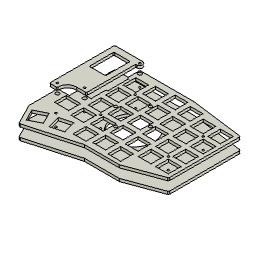
Sofle_pico_v3.4_Acrylic_case v20 (Autodesk Fusion 360 design; units mm, degrees)
Autodesk Fusion 360 part; units mm, degrees
sketch "OLED_raw_import" plane through (0, 0, 0) normal (0, 0, 1) x (1, 0, 0)
  arc A0 (31.596, -60.3171) -> (30.596, -61.3171) centre (30.596, -60.3171) cw
  arc A1 (3.2145, -72.447) -> (2.2145, -71.447) centre (3.2146, -71.4469) cw
  line L0 (31.596, -60.3171) -> (31.596, -7.2074)
  arc A2 (2.1895, -2.4227) -> (3.6899, -0.9223) centre (3.69, -2.4228) cw
  line L1 (2.2145, -71.447) -> (2.1895, -2.4227)
  arc A3 (10.656, -71.447) -> (9.656, -72.447) centre (9.656, -71.447) cw
  line L2 (31.596, -7.2074) -> (32.7961, -7.2077)
  line L3 (3.6899, -0.9224) -> (32.7961, -0.9224)
  line L4 (9.656, -72.447) -> (3.2145, -72.447)
  line L5 (20.846, -61.3171) -> (30.596, -61.3171)
  arc A4 (10.656, -71.447) -> (20.8461, -61.3171) centre (20.7861, -71.447) cw
  arc A5 (32.7961, -0.9224) -> (32.7961, -7.2074) centre (32.7783, -4.0649) cw
  circle A6 centre (32.7961, -4.0649) radius 1.1
  circle A7 centre (25.926, -57.5371) radius 1.1
  circle A8 centre (6.4353, -67.947) radius 1.1
  line L6 (-6.3855, 6.3482) -> (54.659, 6.3482)
  line L7 (54.659, 6.3482) -> (54.659, -85.336)
  line L8 (54.659, -85.336) -> (-6.3855, -85.336)
  line L9 (-6.3855, -85.336) -> (-6.3855, 6.3482)
  line L10 (32.7961, -0.9224) -> (32.7961, 6.3482)
  line L11 (32.7961, -7.2077) -> (54.659, -7.2077)
  line L12 (32.7961, -0.9224) -> (54.659, -1.0458)
  line L13 (3.6899, -0.9224) -> (3.6899, 6.3482)
  line L14 (2.1895, -2.4227) -> (-6.3855, -2.4227)
  line L15 (2.2145, -71.447) -> (-6.3855, -71.447)
  line L16 (3.2145, -72.447) -> (3.2145, -85.336)
  line L17 (9.656, -72.447) -> (9.656, -85.336)
  line L18 (10.656, -71.447) -> (54.659, -71.447)
  line L19 (30.596, -61.3171) -> (30.596, -71.447)
  line L20 (31.596, -60.3171) -> (54.659, -60.3171)
  line L21 (32.7961, -7.2074) -> (32.7961, -60.3171)
  point P0 (33.8961, -4.0649)
  point P1 (27.026, -57.5371)
  point P2 (7.5352, -67.947)
  constraint horizontal L6
  constraint vertical L7
  constraint horizontal L8
  constraint vertical L9
  constraint coincident L6 L10.end
  constraint perpendicular L6 L10
  constraint coincident L7 L11.end
  constraint perpendicular L7 L11
  constraint coincident L7 L12.end
  constraint tangent A5 L12
  constraint coincident L6 L13.end
  constraint perpendicular L6 L13
  constraint coincident L9 L14.end
  constraint perpendicular L9 L14
  constraint coincident L9 L15.end
  constraint perpendicular L9 L15
  constraint coincident L8 L16.end
  constraint perpendicular L8 L16
  constraint coincident L8 L17.end
  constraint perpendicular L8 L17
  constraint coincident L7 L18.end
  constraint perpendicular L7 L18
  constraint coincident L18 L19.end
  constraint perpendicular L18 L19
  constraint coincident L7 L20.end
  constraint perpendicular L7 L20
  constraint coincident L20 L21.end
  constraint perpendicular L20 L21
extrude "Extrude1" add sketch "OLED_raw_import" along normal blind 3 contours A0 A1 L0 A2 L1 A3 L2 L3 L4 L5 A4 A5 makes body 1
sketch "sofle_pico_OLED_v3.4" plane through (0, 0, 3) normal (0, 0, 1) x (-1, 0, 0)
  circle A0 centre (-25.926, 57.5371) radius 1.1
  circle A1 centre (-32.7961, 4.0649) radius 1.1
  circle A2 centre (-6.4353, 67.947) radius 1.1
  line L0 (-3.6899, 0.9224) -> (-3.6899, 0.9223)
  arc A3 (-3.6899, 0.9223) -> (-2.1895, 2.4227) centre (-3.69, 2.4228) ccw
  line L1 (-2.1895, 2.4227) -> (-2.2145, 71.447)
  arc A4 (-2.2145, 71.447) -> (-3.2145, 72.447) centre (-3.2146, 71.4469) ccw
  line L2 (-3.2145, 72.447) -> (-9.656, 72.447)
  arc A5 (-9.656, 72.447) -> (-10.656, 71.447) centre (-9.656, 71.447) ccw
  arc A6 (-20.8461, 61.3171) -> (-10.656, 71.447) centre (-20.7861, 71.447) ccw
  line L3 (-20.8461, 61.3171) -> (-30.596, 61.3171)
  arc A7 (-30.596, 61.3171) -> (-31.596, 60.3171) centre (-30.596, 60.3171) ccw
  line L4 (-31.596, 60.3171) -> (-31.596, 7.2074)
  line L5 (-31.596, 7.2074) -> (-32.7961, 7.2077)
  line L6 (-32.7961, 7.2077) -> (-32.7961, 7.2074)
  arc A8 (-32.7961, 7.2074) -> (-32.7961, 0.9224) centre (-32.7783, 4.0649) ccw
  line L7 (-32.7961, 0.9224) -> (-3.6899, 0.9224)
sketch "keyplate_raw_import" plane through (0, 0, 0) normal (0, 0, 1) x (1, 0, 0)
  arc A0 (64.0629, -94.1892) -> (63.8994, -93.4815) centre (65.4011, -93.5073) cw
  line L0 (64.0629, -94.1892) -> (74.8738, -115.4059)
  arc A1 (91.5088, -0.9271) -> (92.5088, 0.0729) centre (92.5088, -0.9271) cw
  line L1 (150.6703, 0.0729) -> (207.9837, -7.326)
  arc A2 (92.5088, -13.8721) -> (91.5088, -12.8721) centre (92.5088, -12.8721) cw
  line L2 (91.5088, -37.8219) -> (91.5088, -53.3818)
  line L3 (92.5088, -13.8721) -> (93.2959, -13.8721)
  line L4 (63.8994, -63.3988) -> (63.8994, -93.4815)
  line L5 (150.6703, 0.0729) -> (92.5088, 0.0729)
  line L6 (76.596, -62.3988) -> (76.596, -53.3818)
  arc A3 (207.9837, -7.326) -> (209.3199, -8.827) centre (207.8088, -8.827) cw
  line L7 (92.5088, -36.8219) -> (93.2959, -36.8219)
  line L8 (93.2959, -36.8219) -> (93.2959, -13.8721)
  line L9 (91.5088, -53.3818) -> (76.596, -53.3818)
  line L10 (169.7202, -100.6763) -> (208.4142, -86.4036)
  line L11 (209.3199, -8.827) -> (209.3199, -85.0265)
  line L12 (131.6205, -100.6763) -> (169.7202, -100.6763)
  line L13 (91.5088, -0.9271) -> (91.5088, -12.8721)
  line L14 (64.8994, -62.3988) -> (76.596, -62.3988)
  arc A4 (76.6062, -116.1717) -> (74.8738, -115.4059) centre (76.2102, -114.725) cw
  arc A5 (209.3199, -85.0265) -> (208.4142, -86.4037) centre (207.8201, -85.0266) cw
  line L15 (76.6062, -116.1717) -> (131.6205, -100.6763)
  arc A6 (91.5088, -37.8219) -> (92.5088, -36.8219) centre (92.5088, -37.8219) cw
  arc A7 (63.8994, -63.3988) -> (64.8994, -62.3988) centre (64.8994, -63.3988) cw
  line L16 (90.4959, -76.9516) -> (74.896, -76.9516)
  line L17 (74.896, -76.9516) -> (74.896, -63.9517)
  line L18 (74.896, -63.9517) -> (90.4959, -63.9517)
  line L19 (90.4959, -63.9517) -> (90.4959, -76.9516)
  circle A8 centre (188.7852, -27.862) radius 1.1
  circle A9 centre (188.7703, -65.9767) radius 1.1
  circle A10 centre (111.9358, -25.462) radius 1.1
  circle A11 centre (112.0257, -63.4117) radius 1.1
  circle A12 centre (112.5707, -47.3218) radius 1.75
  circle A13 centre (131.6206, -28.272) radius 1.75
  circle A14 centre (131.6206, -66.3717) radius 1.75
  circle A15 centre (150.6704, -47.3218) radius 1.75
  circle A16 centre (86.0859, -86.4815) radius 1.1
  circle A17 centre (94.5059, -3.0695) radius 2.05
  circle A18 centre (87.6359, -56.5418) radius 2.05
  circle A19 centre (68.1451, -66.9517) radius 2.05
  line L20 (110.0457, -22.952) -> (96.0458, -22.952)
  line L21 (96.0458, -22.952) -> (96.0458, -8.9521)
  line L22 (96.0458, -8.9521) -> (110.0457, -8.9521)
  line L23 (110.0457, -8.9521) -> (110.0457, -22.952)
  line L24 (148.1456, -17.952) -> (134.1457, -17.952)
  line L25 (134.1457, -17.952) -> (134.1457, -3.9521)
  line L26 (134.1457, -3.9521) -> (148.1456, -3.9521)
  line L27 (148.1456, -3.9521) -> (148.1456, -17.952)
  line L28 (110.0457, -61.0517) -> (96.0458, -61.0517)
  line L29 (96.0458, -61.0517) -> (96.0458, -47.0518)
  line L30 (96.0458, -47.0518) -> (110.0457, -47.0518)
  line L31 (110.0457, -47.0518) -> (110.0457, -61.0517)
  line L32 (129.0957, -58.5517) -> (115.0957, -58.5517)
  line L33 (115.0957, -58.5517) -> (115.0957, -44.5518)
  line L34 (115.0957, -44.5518) -> (129.0957, -44.5518)
  line L35 (129.0957, -44.5518) -> (129.0957, -58.5517)
  line L36 (148.1456, -75.1016) -> (134.1457, -75.1016)
  line L37 (134.1457, -75.1016) -> (134.1457, -61.1017)
  line L38 (134.1457, -61.1017) -> (148.1456, -61.1017)
  line L39 (148.1456, -61.1017) -> (148.1456, -75.1016)
  line L40 (186.2452, -82.5016) -> (172.2453, -82.5016)
  line L41 (172.2453, -82.5016) -> (172.2453, -68.5017)
  line L42 (172.2453, -68.5017) -> (186.2452, -68.5017)
  line L43 (186.2452, -68.5017) -> (186.2452, -82.5016)
  line L44 (76.2327, -109.2072) -> (69.8768, -96.7332)
  line L45 (69.8768, -96.7332) -> (82.3508, -90.3773)
  line L46 (82.3508, -90.3773) -> (88.7067, -102.8513)
  line L47 (88.7067, -102.8513) -> (76.2327, -109.2072)
  line L48 (108.669, -99.3012) -> (95.1461, -102.9246)
  line L49 (95.1461, -102.9246) -> (91.5227, -89.4018)
  line L50 (91.5227, -89.4018) -> (105.0456, -85.7783)
  line L51 (105.0456, -85.7783) -> (108.669, -99.3012)
  line L52 (205.2951, -44.4018) -> (191.2952, -44.4018)
  line L53 (191.2952, -44.4018) -> (191.2952, -30.4019)
  line L54 (191.2952, -30.4019) -> (205.2951, -30.4019)
  line L55 (205.2951, -30.4019) -> (205.2951, -44.4018)
  line L56 (205.2951, -63.4517) -> (191.2952, -63.4517)
  line L57 (191.2952, -63.4517) -> (191.2952, -49.4518)
  line L58 (191.2952, -49.4518) -> (205.2951, -49.4518)
  line L59 (205.2951, -49.4518) -> (205.2951, -63.4517)
  line L60 (205.2951, -82.5016) -> (191.2952, -82.5016)
  line L61 (191.2952, -82.5016) -> (191.2952, -68.5017)
  line L62 (191.2952, -68.5017) -> (205.2951, -68.5017)
  line L63 (205.2951, -68.5017) -> (205.2951, -82.5016)
  line L64 (167.1953, -20.452) -> (153.1954, -20.452)
  line L65 (153.1954, -20.452) -> (153.1954, -6.4521)
  line L66 (153.1954, -6.4521) -> (167.1953, -6.4521)
  line L67 (167.1953, -6.4521) -> (167.1953, -20.452)
  line L68 (186.2452, -25.352) -> (172.2453, -25.352)
  line L69 (172.2453, -25.352) -> (172.2453, -11.3521)
  line L70 (172.2453, -11.3521) -> (186.2452, -11.3521)
  line L71 (186.2452, -11.3521) -> (186.2452, -25.352)
  line L72 (129.0957, -39.5019) -> (115.0957, -39.5019)
  line L73 (115.0957, -39.5019) -> (115.0957, -25.502)
  line L74 (115.0957, -25.502) -> (129.0957, -25.502)
  line L75 (129.0957, -25.502) -> (129.0957, -39.5019)
  line L76 (167.1953, -39.5019) -> (153.1954, -39.5019)
  line L77 (153.1954, -39.5019) -> (153.1954, -25.502)
  line L78 (153.1954, -25.502) -> (167.1953, -25.502)
  line L79 (167.1953, -25.502) -> (167.1953, -39.5019)
  line L80 (148.1456, -37.0019) -> (134.1457, -37.0019)
  line L81 (134.1457, -37.0019) -> (134.1457, -23.002)
  line L82 (134.1457, -23.002) -> (148.1456, -23.002)
  line L83 (148.1456, -23.002) -> (148.1456, -37.0019)
  line L84 (167.1953, -58.5517) -> (153.1954, -58.5517)
  line L85 (153.1954, -58.5517) -> (153.1954, -44.5518)
  line L86 (153.1954, -44.5518) -> (167.1953, -44.5518)
  line L87 (167.1953, -44.5518) -> (167.1953, -58.5517)
  line L88 (205.2951, -25.352) -> (191.2952, -25.352)
  line L89 (191.2952, -25.352) -> (191.2952, -11.3521)
  line L90 (191.2952, -11.3521) -> (205.2951, -11.3521)
  line L91 (205.2951, -11.3521) -> (205.2951, -25.352)
  line L92 (110.0457, -42.0019) -> (96.0458, -42.0019)
  line L93 (96.0458, -42.0019) -> (96.0458, -28.002)
  line L94 (96.0458, -28.002) -> (110.0457, -28.002)
  line L95 (110.0457, -28.002) -> (110.0457, -42.0019)
  line L96 (167.1953, -96.6515) -> (153.1954, -96.6515)
  line L97 (153.1954, -96.6515) -> (153.1954, -82.6516)
  line L98 (153.1954, -82.6516) -> (167.1953, -82.6516)
  line L99 (167.1953, -82.6516) -> (167.1953, -96.6515)
  line L100 (186.2452, -44.4018) -> (172.2453, -44.4018)
  line L101 (172.2453, -44.4018) -> (172.2453, -30.4019)
  line L102 (172.2453, -30.4019) -> (186.2452, -30.4019)
  line L103 (186.2452, -30.4019) -> (186.2452, -44.4018)
  line L104 (167.1953, -77.6016) -> (153.1954, -77.6016)
  line L105 (153.1954, -77.6016) -> (153.1954, -63.6017)
  line L106 (153.1954, -63.6017) -> (167.1953, -63.6017)
  line L107 (167.1953, -63.6017) -> (167.1953, -77.6016)
  line L108 (186.2452, -63.4517) -> (172.2453, -63.4517)
  line L109 (172.2453, -63.4517) -> (172.2453, -49.4518)
  line L110 (172.2453, -49.4518) -> (186.2452, -49.4518)
  line L111 (186.2452, -49.4518) -> (186.2452, -63.4517)
  line L112 (148.1456, -94.1515) -> (134.1457, -94.1515)
  line L113 (134.1457, -94.1515) -> (134.1457, -80.1516)
  line L114 (134.1457, -80.1516) -> (148.1456, -80.1516)
  line L115 (148.1456, -80.1516) -> (148.1456, -94.1515)
  line L116 (148.1456, -56.0518) -> (134.1457, -56.0518)
  line L117 (134.1457, -56.0518) -> (134.1457, -42.0519)
  line L118 (134.1457, -42.0519) -> (148.1456, -42.0519)
  line L119 (148.1456, -42.0519) -> (148.1456, -56.0518)
  line L120 (129.0957, -20.452) -> (115.0957, -20.452)
  line L121 (115.0957, -20.452) -> (115.0957, -6.4521)
  line L122 (115.0957, -6.4521) -> (129.0957, -6.4521)
  line L123 (129.0957, -6.4521) -> (129.0957, -20.452)
  line L124 (129.0957, -77.6016) -> (115.0957, -77.6016)
  line L125 (115.0957, -77.6016) -> (115.0957, -63.6017)
  line L126 (115.0957, -63.6017) -> (129.0957, -63.6017)
  line L127 (129.0957, -63.6017) -> (129.0957, -77.6016)
  line L128 (129.0957, -96.6515) -> (115.0957, -96.6515)
  line L129 (115.0957, -96.6515) -> (115.0957, -82.6516)
  line L130 (115.0957, -82.6516) -> (129.0957, -82.6516)
  line L131 (129.0957, -82.6516) -> (129.0957, -96.6515)
  line L132 (110.0457, -80.1016) -> (96.0458, -80.1016)
  line L133 (96.0458, -80.1016) -> (96.0458, -66.1017)
  line L134 (96.0458, -66.1017) -> (110.0457, -66.1017)
  line L135 (110.0457, -66.1017) -> (110.0457, -80.1016)
  line L136 (58.3963, 5.3223) -> (215.5932, 5.3223)
  line L137 (215.5932, 5.3223) -> (215.5932, -121.9444)
  line L138 (215.5932, -121.9444) -> (58.3963, -121.9444)
  line L139 (58.3963, -121.9444) -> (58.3963, 5.3223)
  line L140 (76.6062, -116.1717) -> (76.6062, -121.9444)
  line L141 (131.6205, -100.6763) -> (131.6205, -121.9444)
  line L142 (209.3199, -8.827) -> (215.5932, -8.827)
  line L143 (207.9837, -7.326) -> (207.9837, 5.3223)
  line L144 (91.5088, -12.8721) -> (58.3963, -12.8721)
  line L145 (92.5088, 0.0729) -> (92.5088, 5.3223)
  line L146 (76.596, -53.3818) -> (58.3963, -53.3818)
  line L147 (209.3199, -85.0265) -> (215.5932, -85.0265)
  line L148 (208.4142, -86.4037) -> (215.5932, -86.4037)
  line L149 (169.7202, -100.6763) -> (169.7202, -121.9444)
  line L150 (208.4142, -86.4036) -> (208.4142, -121.9444)
  point P0 (189.8851, -27.862)
  point P1 (189.8702, -65.9767)
  point P2 (113.0358, -25.462)
  point P3 (113.1257, -63.4117)
  point P4 (114.3207, -47.3218)
  point P5 (133.3706, -28.272)
  point P6 (133.3706, -66.3717)
  point P7 (152.4204, -47.3218)
  point P8 (87.1859, -86.4815)
  point P9 (96.5559, -3.0695)
  point P10 (89.6859, -56.5418)
  point P11 (70.1951, -66.9517)
  constraint horizontal L136
  constraint vertical L137
  constraint horizontal L138
  constraint vertical L139
  constraint coincident L138 L140.end
  constraint perpendicular L138 L140
  constraint coincident L138 L141.end
  constraint perpendicular L138 L141
  constraint coincident L137 L142.end
  constraint perpendicular L137 L142
  constraint coincident L136 L143.end
  constraint perpendicular L136 L143
  constraint coincident L139 L144.end
  constraint perpendicular L139 L144
  constraint coincident L136 L145.end
  constraint perpendicular L136 L145
  constraint coincident L139 L146.end
  constraint perpendicular L139 L146
  constraint coincident L137 L147.end
  constraint perpendicular L137 L147
  constraint coincident L137 L148.end
  constraint perpendicular L137 L148
  constraint coincident L138 L149.end
  constraint perpendicular L138 L149
  constraint coincident L138 L150.end
  constraint perpendicular L138 L150
extrude "Extrude2" add sketch "keyplate_raw_import" along normal blind 3 separate body contours A0 L0 A1 L1 A2 L2 L3 L4 L5 L6 A3 L7 L8 L9 L10 L11 L12 L13 L14 A4 A5 L15 A6 A7 makes body 2
sketch "sofle_pico_keyplate_v3.4" plane through (0, 0, 3) normal (0, 0, 1) x (-1, 0, 0)
  line L0 (-74.896, 63.9517) -> (-90.4959, 63.9517)
  line L1 (-90.4959, 63.9517) -> (-90.4959, 76.9516)
  line L2 (-90.4959, 76.9516) -> (-74.896, 76.9516)
  line L3 (-74.896, 76.9516) -> (-74.896, 63.9517)
  circle A0 centre (-131.6206, 66.3717) radius 1.75
  circle A1 centre (-188.7852, 27.862) radius 1.1
  circle A2 centre (-188.7703, 65.9767) radius 1.1
  circle A3 centre (-111.9358, 25.462) radius 1.1
  circle A4 centre (-112.0257, 63.4117) radius 1.1
  line L4 (-172.2453, 11.3521) -> (-186.2452, 11.3521)
  line L5 (-186.2452, 11.3521) -> (-186.2452, 25.352)
  line L6 (-186.2452, 25.352) -> (-172.2453, 25.352)
  line L7 (-172.2453, 25.352) -> (-172.2453, 11.3521)
  circle A5 centre (-112.5707, 47.3218) radius 1.75
  circle A6 centre (-131.6206, 28.272) radius 1.75
  line L8 (-82.3508, 90.3773) -> (-88.7067, 102.8513)
  line L9 (-88.7067, 102.8513) -> (-76.2327, 109.2072)
  line L10 (-76.2327, 109.2072) -> (-69.8768, 96.7332)
  line L11 (-69.8768, 96.7332) -> (-82.3508, 90.3773)
  line L12 (-91.5227, 89.4018) -> (-105.0456, 85.7783)
  line L13 (-105.0456, 85.7783) -> (-108.669, 99.3012)
  line L14 (-108.669, 99.3012) -> (-95.1461, 102.9246)
  line L15 (-95.1461, 102.9246) -> (-91.5227, 89.4018)
  line L16 (-134.1457, 3.9521) -> (-148.1456, 3.9521)
  line L17 (-148.1456, 3.9521) -> (-148.1456, 17.952)
  line L18 (-148.1456, 17.952) -> (-134.1457, 17.952)
  line L19 (-134.1457, 17.952) -> (-134.1457, 3.9521)
  line L20 (-96.0458, 8.9521) -> (-110.0457, 8.9521)
  line L21 (-110.0457, 8.9521) -> (-110.0457, 22.952)
  line L22 (-110.0457, 22.952) -> (-96.0458, 22.952)
  line L23 (-96.0458, 22.952) -> (-96.0458, 8.9521)
  circle A7 centre (-68.1451, 66.9517) radius 2.05
  circle A8 centre (-87.6359, 56.5418) radius 2.05
  circle A9 centre (-94.5059, 3.0695) radius 2.05
  circle A10 centre (-86.0859, 86.4815) radius 1.1
  circle A11 centre (-150.6704, 47.3218) radius 1.75
  line L24 (-96.0458, 28.002) -> (-110.0457, 28.002)
  line L25 (-110.0457, 28.002) -> (-110.0457, 42.0019)
  line L26 (-110.0457, 42.0019) -> (-96.0458, 42.0019)
  line L27 (-96.0458, 42.0019) -> (-96.0458, 28.002)
  line L28 (-172.2453, 68.5017) -> (-186.2452, 68.5017)
  line L29 (-186.2452, 68.5017) -> (-186.2452, 82.5016)
  line L30 (-186.2452, 82.5016) -> (-172.2453, 82.5016)
  line L31 (-172.2453, 82.5016) -> (-172.2453, 68.5017)
  line L32 (-134.1457, 61.1017) -> (-148.1456, 61.1017)
  line L33 (-148.1456, 61.1017) -> (-148.1456, 75.1016)
  line L34 (-148.1456, 75.1016) -> (-134.1457, 75.1016)
  line L35 (-134.1457, 75.1016) -> (-134.1457, 61.1017)
  line L36 (-96.0458, 47.0518) -> (-110.0457, 47.0518)
  line L37 (-110.0457, 47.0518) -> (-110.0457, 61.0517)
  line L38 (-110.0457, 61.0517) -> (-96.0458, 61.0517)
  line L39 (-96.0458, 61.0517) -> (-96.0458, 47.0518)
  line L40 (-115.0957, 44.5518) -> (-129.0957, 44.5518)
  line L41 (-129.0957, 44.5518) -> (-129.0957, 58.5517)
  line L42 (-129.0957, 58.5517) -> (-115.0957, 58.5517)
  line L43 (-115.0957, 58.5517) -> (-115.0957, 44.5518)
  line L44 (-115.0957, 25.502) -> (-129.0957, 25.502)
  line L45 (-129.0957, 25.502) -> (-129.0957, 39.5019)
  line L46 (-129.0957, 39.5019) -> (-115.0957, 39.5019)
  line L47 (-115.0957, 39.5019) -> (-115.0957, 25.502)
  line L48 (-153.1954, 6.4521) -> (-167.1953, 6.4521)
  line L49 (-167.1953, 6.4521) -> (-167.1953, 20.452)
  line L50 (-167.1953, 20.452) -> (-153.1954, 20.452)
  line L51 (-153.1954, 20.452) -> (-153.1954, 6.4521)
  line L52 (-134.1457, 80.1516) -> (-148.1456, 80.1516)
  line L53 (-148.1456, 80.1516) -> (-148.1456, 94.1515)
  line L54 (-148.1456, 94.1515) -> (-134.1457, 94.1515)
  line L55 (-134.1457, 94.1515) -> (-134.1457, 80.1516)
  line L56 (-191.2952, 68.5017) -> (-205.2951, 68.5017)
  line L57 (-205.2951, 68.5017) -> (-205.2951, 82.5016)
  line L58 (-205.2951, 82.5016) -> (-191.2952, 82.5016)
  line L59 (-191.2952, 82.5016) -> (-191.2952, 68.5017)
  line L60 (-191.2952, 30.4019) -> (-205.2951, 30.4019)
  line L61 (-205.2951, 30.4019) -> (-205.2951, 44.4018)
  line L62 (-205.2951, 44.4018) -> (-191.2952, 44.4018)
  line L63 (-191.2952, 44.4018) -> (-191.2952, 30.4019)
  line L64 (-191.2952, 49.4518) -> (-205.2951, 49.4518)
  line L65 (-205.2951, 49.4518) -> (-205.2951, 63.4517)
  line L66 (-205.2951, 63.4517) -> (-191.2952, 63.4517)
  line L67 (-191.2952, 63.4517) -> (-191.2952, 49.4518)
  line L68 (-134.1457, 42.0519) -> (-148.1456, 42.0519)
  line L69 (-148.1456, 42.0519) -> (-148.1456, 56.0518)
  line L70 (-148.1456, 56.0518) -> (-134.1457, 56.0518)
  line L71 (-134.1457, 56.0518) -> (-134.1457, 42.0519)
  line L72 (-191.2952, 11.3521) -> (-205.2951, 11.3521)
  line L73 (-205.2951, 11.3521) -> (-205.2951, 25.352)
  line L74 (-205.2951, 25.352) -> (-191.2952, 25.352)
  line L75 (-191.2952, 25.352) -> (-191.2952, 11.3521)
  line L76 (-153.1954, 44.5518) -> (-167.1953, 44.5518)
  line L77 (-167.1953, 44.5518) -> (-167.1953, 58.5517)
  line L78 (-167.1953, 58.5517) -> (-153.1954, 58.5517)
  line L79 (-153.1954, 58.5517) -> (-153.1954, 44.5518)
  line L80 (-134.1457, 23.002) -> (-148.1456, 23.002)
  line L81 (-148.1456, 23.002) -> (-148.1456, 37.0019)
  line L82 (-148.1456, 37.0019) -> (-134.1457, 37.0019)
  line L83 (-134.1457, 37.0019) -> (-134.1457, 23.002)
  line L84 (-153.1954, 25.502) -> (-167.1953, 25.502)
  line L85 (-167.1953, 25.502) -> (-167.1953, 39.5019)
  line L86 (-167.1953, 39.5019) -> (-153.1954, 39.5019)
  line L87 (-153.1954, 39.5019) -> (-153.1954, 25.502)
  line L88 (-172.2453, 49.4518) -> (-186.2452, 49.4518)
  line L89 (-186.2452, 49.4518) -> (-186.2452, 63.4517)
  line L90 (-186.2452, 63.4517) -> (-172.2453, 63.4517)
  line L91 (-172.2453, 63.4517) -> (-172.2453, 49.4518)
  line L92 (-153.1954, 63.6017) -> (-167.1953, 63.6017)
  line L93 (-167.1953, 63.6017) -> (-167.1953, 77.6016)
  line L94 (-167.1953, 77.6016) -> (-153.1954, 77.6016)
  line L95 (-153.1954, 77.6016) -> (-153.1954, 63.6017)
  line L96 (-153.1954, 82.6516) -> (-167.1953, 82.6516)
  line L97 (-167.1953, 82.6516) -> (-167.1953, 96.6515)
  line L98 (-167.1953, 96.6515) -> (-153.1954, 96.6515)
  line L99 (-153.1954, 96.6515) -> (-153.1954, 82.6516)
  line L100 (-172.2453, 30.4019) -> (-186.2452, 30.4019)
  line L101 (-186.2452, 30.4019) -> (-186.2452, 44.4018)
  line L102 (-186.2452, 44.4018) -> (-172.2453, 44.4018)
  line L103 (-172.2453, 44.4018) -> (-172.2453, 30.4019)
  line L104 (-96.0458, 66.1017) -> (-110.0457, 66.1017)
  line L105 (-110.0457, 66.1017) -> (-110.0457, 80.1016)
  line L106 (-110.0457, 80.1016) -> (-96.0458, 80.1016)
  line L107 (-96.0458, 80.1016) -> (-96.0458, 66.1017)
  line L108 (-115.0957, 82.6516) -> (-129.0957, 82.6516)
  line L109 (-129.0957, 82.6516) -> (-129.0957, 96.6515)
  line L110 (-129.0957, 96.6515) -> (-115.0957, 96.6515)
  line L111 (-115.0957, 96.6515) -> (-115.0957, 82.6516)
  line L112 (-115.0957, 6.4521) -> (-129.0957, 6.4521)
  line L113 (-129.0957, 6.4521) -> (-129.0957, 20.452)
  line L114 (-129.0957, 20.452) -> (-115.0957, 20.452)
  line L115 (-115.0957, 20.452) -> (-115.0957, 6.4521)
  line L116 (-115.0957, 63.6017) -> (-129.0957, 63.6017)
  line L117 (-129.0957, 63.6017) -> (-129.0957, 77.6016)
  line L118 (-129.0957, 77.6016) -> (-115.0957, 77.6016)
  line L119 (-115.0957, 77.6016) -> (-115.0957, 63.6017)
  line L120 (-76.6062, 116.1717) -> (-131.6205, 100.6763)
  line L121 (-131.6205, 100.6763) -> (-169.7202, 100.6763)
  line L122 (-169.7202, 100.6763) -> (-208.4142, 86.4036)
  line L123 (-208.4142, 86.4036) -> (-208.4142, 86.4037)
  arc A12 (-208.4142, 86.4037) -> (-209.3199, 85.0265) centre (-207.8201, 85.0266) ccw
  line L124 (-209.3199, 85.0265) -> (-209.3199, 8.827)
  arc A13 (-209.3199, 8.827) -> (-207.9837, 7.326) centre (-207.8088, 8.827) ccw
  line L125 (-207.9837, 7.326) -> (-150.6703, -0.0729)
  line L126 (-150.6703, -0.0729) -> (-92.5088, -0.0729)
  arc A14 (-92.5088, -0.0729) -> (-91.5088, 0.9271) centre (-92.5088, 0.9271) ccw
  line L127 (-91.5088, 0.9271) -> (-91.5088, 12.8721)
  arc A15 (-91.5088, 12.8721) -> (-92.5088, 13.8721) centre (-92.5088, 12.8721) ccw
  line L128 (-92.5088, 13.8721) -> (-93.2959, 13.8721)
  line L129 (-93.2959, 13.8721) -> (-93.2959, 36.8219)
  line L130 (-93.2959, 36.8219) -> (-92.5088, 36.8219)
  arc A16 (-92.5088, 36.8219) -> (-91.5088, 37.8219) centre (-92.5088, 37.8219) ccw
  line L131 (-91.5088, 37.8219) -> (-91.5088, 53.3818)
  line L132 (-91.5088, 53.3818) -> (-76.596, 53.3818)
  line L133 (-76.596, 53.3818) -> (-76.596, 62.3988)
  line L134 (-76.596, 62.3988) -> (-64.8994, 62.3988)
  arc A17 (-64.8994, 62.3988) -> (-63.8994, 63.3988) centre (-64.8994, 63.3988) ccw
  line L135 (-63.8994, 63.3988) -> (-63.8994, 93.4815)
  arc A18 (-63.8994, 93.4815) -> (-64.0629, 94.1892) centre (-65.4011, 93.5073) ccw
  line L136 (-64.0629, 94.1892) -> (-74.8738, 115.4059)
  arc A19 (-74.8738, 115.4059) -> (-76.6062, 116.1717) centre (-76.2102, 114.725) ccw
sketch "backplate_raw_import" plane through (0, 0, 0) normal (0, 0, 1) x (1, 0, 0)
  arc A0 (-169.4719, -112.9235) -> (-169.6354, -112.2158) centre (-168.1337, -112.2416) cw
  line L0 (-82.8644, -18.6614) -> (-25.551, -26.0603)
  arc A1 (-24.2149, -103.7608) -> (-25.1206, -105.138) centre (-25.7147, -103.7608) cw
  line L1 (-101.9143, -119.4107) -> (-63.8146, -119.4107)
  arc A2 (-25.551, -26.0603) -> (-24.2149, -27.5613) centre (-25.7259, -27.5613) cw
  line L2 (-82.8644, -18.6614) -> (-168.135, -18.6614)
  arc A3 (-156.9286, -134.9061) -> (-158.661, -134.1403) centre (-157.3245, -133.4594) cw
  line L3 (-169.4719, -112.9235) -> (-158.661, -134.1403)
  arc A4 (-169.6354, -20.1617) -> (-168.135, -18.6613) centre (-168.1349, -20.1618) cw
  line L4 (-169.6354, -20.1617) -> (-169.6354, -112.2158)
  line L5 (-24.2149, -27.5613) -> (-24.2149, -103.7608)
  line L6 (-63.8146, -119.4107) -> (-25.1206, -105.138)
  line L7 (-156.9286, -134.9061) -> (-101.9143, -119.4107)
  circle A5 centre (-44.7496, -46.5963) radius 1.1
  circle A6 centre (-44.7645, -84.711) radius 1.1
  circle A7 centre (-121.5989, -44.1963) radius 1.1
  circle A8 centre (-121.509, -82.146) radius 1.1
  circle A9 centre (-101.9142, -66.0562) radius 22.4998
  circle A10 centre (-147.4489, -105.2159) radius 1.1
  circle A11 centre (-139.0288, -21.8039) radius 1.1
  circle A12 centre (-145.8989, -75.2761) radius 1.1
  circle A13 centre (-165.3896, -85.686) radius 1.1
  line L8 (-175.6509, -14.2608) -> (-18.4347, -14.2608)
  line L9 (-18.4347, -14.2608) -> (-18.4347, -140.8686)
  line L10 (-18.4347, -140.8686) -> (-175.6509, -140.8686)
  line L11 (-175.6509, -140.8686) -> (-175.6509, -14.2608)
  line L12 (-82.8644, -18.6614) -> (-82.8644, -14.2608)
  line L13 (-168.135, -18.6614) -> (-168.135, -14.2608)
  line L14 (-168.135, -18.6613) -> (-82.8644, -18.6614)
  point P0 (-43.6496, -46.5963)
  point P1 (-43.6645, -84.711)
  point P2 (-120.499, -44.1963)
  point P3 (-120.4091, -82.146)
  point P4 (-79.4144, -66.0562)
  point P5 (-146.3489, -105.2159)
  point P6 (-137.9288, -21.8039)
  point P7 (-144.7989, -75.2761)
  point P8 (-164.2896, -85.686)
  constraint horizontal L8
  constraint vertical L9
  constraint horizontal L10
  constraint vertical L11
  constraint coincident L8 L12.end
  constraint perpendicular L8 L12
  constraint coincident L8 L13.end
  constraint perpendicular L8 L13
extrude "Extrude3" add sketch "backplate_raw_import" along normal blind 3 separate body contours A0 L0 A1 L1 A2 L2 A3 L3 A4 L4 L5 L6 L7 L14 makes body 3
sketch "sofle_pico_backplate_v3.4" plane through (0, 0, 3) normal (0, 0, 1) x (-1, 0, 0)
  circle A0 centre (44.7645, 84.711) radius 1.1
  circle A1 centre (101.9142, 66.0562) radius 22.4998
  circle A2 centre (44.7496, 46.5963) radius 1.1
  circle A3 centre (145.8989, 75.2761) radius 1.1
  circle A4 centre (121.509, 82.146) radius 1.1
  circle A5 centre (121.5989, 44.1963) radius 1.1
  circle A6 centre (139.0288, 21.8039) radius 1.1
  circle A7 centre (165.3896, 85.686) radius 1.1
  circle A8 centre (147.4489, 105.2159) radius 1.1
  line L0 (82.8644, 18.6614) -> (168.135, 18.6614)
  line L1 (168.135, 18.6614) -> (168.135, 18.6613)
  arc A9 (168.135, 18.6613) -> (169.6354, 20.1617) centre (168.1349, 20.1618) ccw
  line L2 (169.6354, 20.1617) -> (169.6354, 112.2158)
  arc A10 (169.6354, 112.2158) -> (169.4719, 112.9235) centre (168.1337, 112.2416) ccw
  line L3 (169.4719, 112.9235) -> (158.661, 134.1403)
  arc A11 (158.661, 134.1403) -> (156.9286, 134.9061) centre (157.3245, 133.4594) ccw
  line L4 (156.9286, 134.9061) -> (101.9143, 119.4107)
  line L5 (101.9143, 119.4107) -> (63.8146, 119.4107)
  line L6 (63.8146, 119.4107) -> (25.1206, 105.138)
  arc A12 (25.1206, 105.138) -> (24.2149, 103.7608) centre (25.7147, 103.7608) ccw
  line L7 (24.2149, 103.7608) -> (24.2149, 27.5613)
  arc A13 (24.2149, 27.5613) -> (25.551, 26.0603) centre (25.7259, 27.5613) ccw
  line L8 (25.551, 26.0603) -> (82.8644, 18.6614)
move_body "Move1" bodies 3 to x (1, 0, 0) y (0, 1, 0) z (0, 0, 1) at (233.5348, 18.7343, -3)
move_body "Move2" bodies 3 to x (1, 0, 0) y (0, 1, 0) z (0, 0, 1) at (0, 0, -10)
move_body "Move3" bodies 1 to x (1, 0, 0) y (0, 1, 0) z (0, 0, 1) at (61.7099, 0.9953, 0)
move_body "Move4" bodies 1 to x (1, 0, 0) y (0, 1, 0) z (0, 0, 1) at (0, 0, 10)
sketch "OLED_with_Windows_raw_import" plane through (0, 0, 0) normal (0, 0, 1) x (1, 0, 0)
  arc A0 (-28.3022, 23.7448) -> (-29.3022, 22.7449) centre (-29.3022, 23.7448) cw
  line L0 (-56.2084, 83.1396) -> (-27.1022, 83.1396)
  line L1 (-28.3022, 23.7448) -> (-28.3022, 76.8545)
  arc A1 (-27.1022, 76.8542) -> (-27.1022, 83.1399) centre (-27.1022, 79.997) cw
  arc A2 (-57.7088, 81.6392) -> (-56.2084, 83.1396) centre (-56.2083, 81.6391) cw
  arc A3 (-49.2423, 12.6149) -> (-50.2423, 11.6149) centre (-50.2423, 12.6149) cw
  line L2 (-50.2423, 11.6149) -> (-56.6838, 11.6149)
  arc A4 (-56.6838, 11.6149) -> (-57.6837, 12.6149) centre (-56.6837, 12.6149) cw
  line L3 (-39.0521, 22.7449) -> (-29.3022, 22.7449)
  line L4 (-57.6837, 12.6149) -> (-57.7088, 81.6392)
  line L5 (-28.3022, 76.8545) -> (-27.1022, 76.8542)
  arc A5 (-49.2423, 12.6149) -> (-39.0521, 22.7449) centre (-39.1121, 12.6149) cw
  line L6 (-33.9697, 76.3245) -> (-51.7595, 76.3245)
  line L7 (-51.7595, 76.3245) -> (-51.7595, 49.3547)
  line L8 (-51.7595, 49.3547) -> (-33.9697, 49.3547)
  line L9 (-33.9697, 49.3547) -> (-33.9697, 76.3245)
  line L10 (-33.9697, 66.1745) -> (-51.7595, 66.1745)
  line L11 (-51.7595, 66.1745) -> (-51.7595, 39.1747)
  line L12 (-51.7595, 39.1747) -> (-33.9697, 39.1747)
  line L13 (-33.9697, 39.1747) -> (-33.9697, 66.1745)
  circle A6 centre (-27.1022, 79.997) radius 1.1
  circle A7 centre (-33.9722, 26.5248) radius 1.1
  circle A8 centre (-53.463, 16.1149) radius 1.1
  line L14 (-61.4226, 86.3149) -> (-21.1208, 86.3149)
  line L15 (-21.1208, 86.3149) -> (-21.1208, 4.8492)
  line L16 (-21.1208, 4.8492) -> (-61.4226, 4.8492)
  line L17 (-61.4226, 4.8492) -> (-61.4226, 86.3149)
  circle A9 centre (-27.1022, 79.997) radius 3.1429
  point P0 (-26.0022, 79.997)
  point P1 (-32.8722, 26.5248)
  point P2 (-52.363, 16.1149)
  constraint horizontal L14
  constraint vertical L15
  constraint horizontal L16
  constraint vertical L17
  constraint concentric A1 A9
  constraint coincident A1.end A9
extrude "Extrude4" add sketch "OLED_with_Windows_raw_import" along normal blind 3 separate body contours A1 A9 makes body 4
extrude "Extrude5" add sketch "OLED_with_Windows_raw_import" along normal blind 3 contours A0 L0 L1 A1 A2 A3 L2 A4 L3 L4 L5 A5 A9 | L8 L11 L12 L13 bodies 4
extrude "Extrude6" add sketch "OLED_with_Windows_raw_import" along normal blind 3 separate body contours A1 A9 makes body 5
extrude "Extrude7" add sketch "OLED_with_Windows_raw_import" along normal blind 3 contours A0 L0 L1 A1 A2 A3 L2 A4 L3 L4 L5 A5 A9 | L6 L7 L9 L10 bodies 5
fillet "Fillet1" radius 1 8 edges at (-33.9697, 49.3547, 1.5) (-51.7595, 49.3547, 1.5) (-33.9697, 76.3245, 1.5) (-51.7595, 76.3245, 1.5) (-33.9697, 66.1745, 1.5) (-51.7595, 66.1745, 1.5) (-33.9697, 39.1747, 1.5) (-51.7595, 39.1747, 1.5) on bodies 4 5
move_body "Move5" bodies 5 to x (1, 0, 0) y (0, 1, 0) z (0, 0, 1) at (121.6082, -83.0666, 13)
move_body "Move6" bodies 5 to x (1, 0, 0) y (0, 1, 0) z (0, 0, 1) at (0, 0, -3)
move_body "Move7" bodies 4 to x (1, 0, 0) y (0, 1, 0) z (0, 0, 1) at (121.6082, -83.0666, 13)
move_body "Move8" bodies 4 to x (1, 0, 0) y (0, 1, 0) z (0, 0, 1) at (0, 0, -3)
move_body "Move9" bodies 5 to x (1, 0, 0) y (0, 1, 0) z (0, 0, 1) at (-40, 0, 0)
sketch "Sketch8" plane through (0, 0, 0) normal (0, 0, 1) x (1, 0, 0)
  spline S0 degree 2 poles (25.8405, 6.1153) (25.8405, 5.6975) (25.9983, 5.3447) knots 0 0 0 1 1 1
  spline S1 degree 2 poles (25.9983, 5.3447) (26.1561, 4.9919) (26.4253, 4.732) knots 0 0 0 1 1 1
  spline S2 degree 2 poles (26.4253, 4.732) (26.6946, 4.472) (27.0474, 4.3235) knots 0 0 0 1 1 1
  spline S3 degree 2 poles (27.0474, 4.3235) (27.4094, 4.1842) (27.8086, 4.1842) knots 0 0 0 1 1 1
  spline S4 degree 2 poles (27.8086, 4.1842) (28.2078, 4.1842) (28.5606, 4.3235) knots 0 0 0 1 1 1
  spline S5 degree 2 poles (28.5606, 4.3235) (28.9227, 4.472) (29.1919, 4.732) knots 0 0 0 1 1 1
  spline S6 degree 2 poles (29.1919, 4.732) (29.4704, 4.9919) (29.6283, 5.3447) knots 0 0 0 1 1 1
  spline S7 degree 2 poles (29.6283, 5.3447) (29.7861, 5.6975) (29.7861, 6.1153) knots 0 0 0 1 1 1
  spline S8 degree 2 poles (29.7861, 6.1153) (29.7861, 6.533) (29.6283, 6.8858) knots 0 0 0 1 1 1
  spline S9 degree 2 poles (29.6283, 6.8858) (29.4704, 7.2386) (29.1919, 7.4985) knots 0 0 0 1 1 1
  spline S10 degree 2 poles (29.1919, 7.4985) (28.9227, 7.7585) (28.5606, 7.8978) knots 0 0 0 1 1 1
  spline S11 degree 2 poles (28.5606, 7.8978) (28.2078, 8.0463) (27.8086, 8.0463) knots 0 0 0 1 1 1
  spline S12 degree 2 poles (27.8086, 8.0463) (27.4094, 8.0463) (27.0474, 7.8978) knots 0 0 0 1 1 1
  spline S13 degree 2 poles (27.0474, 7.8978) (26.6946, 7.7585) (26.4253, 7.4985) knots 0 0 0 1 1 1
  spline S14 degree 2 poles (26.4253, 7.4985) (26.1561, 7.2386) (25.9983, 6.8858) knots 0 0 0 1 1 1
  spline S15 degree 2 poles (25.9983, 6.8858) (25.8405, 6.533) (25.8405, 6.1153) knots 0 0 0 1 1 1
  spline S16 degree 2 poles (23.9373, 6.1153) (23.9373, 6.8951) (24.2251, 7.5635) knots 0 0 0 1 1 1
  spline S17 degree 2 poles (24.2251, 7.5635) (24.5129, 8.2413) (25.0235, 8.7426) knots 0 0 0 1 1 1
  spline S18 degree 2 poles (25.0235, 8.7426) (25.5341, 9.2439) (26.2397, 9.5224) knots 0 0 0 1 1 1
  spline S19 degree 2 poles (26.2397, 9.5224) (26.9545, 9.8102) (27.8086, 9.8102) knots 0 0 0 1 1 1
  spline S20 degree 2 poles (27.8086, 9.8102) (28.6535, 9.8102) (29.3683, 9.5224) knots 0 0 0 1 1 1
  spline S21 degree 2 poles (29.3683, 9.5224) (30.0832, 9.2439) (30.5938, 8.7426) knots 0 0 0 1 1 1
  spline S22 degree 2 poles (30.5938, 8.7426) (31.1137, 8.2413) (31.4015, 7.5635) knots 0 0 0 1 1 1
  spline S23 degree 2 poles (31.4015, 7.5635) (31.6893, 6.8951) (31.6893, 6.1153) knots 0 0 0 1 1 1
  spline S24 degree 2 poles (31.6893, 6.1153) (31.6893, 5.3354) (31.4015, 4.6577) knots 0 0 0 1 1 1
  spline S25 degree 2 poles (31.4015, 4.6577) (31.1137, 3.9893) (30.5938, 3.4879) knots 0 0 0 1 1 1
  spline S26 degree 2 poles (30.5938, 3.4879) (30.0832, 2.9866) (29.3683, 2.6988) knots 0 0 0 1 1 1
  spline S27 degree 2 poles (29.3683, 2.6988) (28.6535, 2.4203) (27.8086, 2.4203) knots 0 0 0 1 1 1
  spline S28 degree 2 poles (27.8086, 2.4203) (26.9545, 2.4203) (26.2397, 2.6988) knots 0 0 0 1 1 1
  spline S29 degree 2 poles (26.2397, 2.6988) (25.5341, 2.9866) (25.0235, 3.4879) knots 0 0 0 1 1 1
  spline S30 degree 2 poles (25.0235, 3.4879) (24.5129, 3.9893) (24.2251, 4.6577) knots 0 0 0 1 1 1
  spline S31 degree 2 poles (24.2251, 4.6577) (23.9373, 5.3354) (23.9373, 6.1153) knots 0 0 0 1 1 1
  line L0 (34.0009, 7.3779) -> (35.1336, 4.9362)
  line L1 (35.1336, 4.9362) -> (36.2848, 7.3779)
  line L2 (36.2848, 7.3779) -> (38.1601, 7.3779)
  line L3 (38.1601, 7.3779) -> (35.6813, 2.6153)
  line L4 (35.6813, 2.6153) -> (34.558, 2.6153)
  line L5 (34.558, 2.6153) -> (32.107, 7.3779)
  line L6 (32.107, 7.3779) -> (34.0009, 7.3779)
  spline S32 degree 2 poles (40.2954, 5.0105) (40.2954, 4.7784) (40.3789, 4.5741) knots 0 0 0 1 1 1
  spline S33 degree 2 poles (40.3789, 4.5741) (40.4625, 4.3792) (40.6017, 4.2306) knots 0 0 0 1 1 1
  spline S34 degree 2 poles (40.6017, 4.2306) (40.7503, 4.0821) (40.9452, 3.9985) knots 0 0 0 1 1 1
  spline S35 degree 2 poles (40.9452, 3.9985) (41.1495, 3.915) (41.3816, 3.915) knots 0 0 0 1 1 1
  spline S36 degree 2 poles (41.3816, 3.915) (41.6044, 3.915) (41.7994, 3.9985) knots 0 0 0 1 1 1
  spline S37 degree 2 poles (41.7994, 3.9985) (42.0036, 4.0821) (42.1429, 4.2306) knots 0 0 0 1 1 1
  spline S38 degree 2 poles (42.1429, 4.2306) (42.2914, 4.3792) (42.3749, 4.5741) knots 0 0 0 1 1 1
  spline S39 degree 2 poles (42.3749, 4.5741) (42.4678, 4.7691) (42.4678, 4.9919) knots 0 0 0 1 1 1
  spline S40 degree 2 poles (42.4678, 4.9919) (42.4678, 5.2147) (42.3749, 5.4097) knots 0 0 0 1 1 1
  spline S41 degree 2 poles (42.3749, 5.4097) (42.2914, 5.6139) (42.1429, 5.7625) knots 0 0 0 1 1 1
  spline S42 degree 2 poles (42.1429, 5.7625) (42.0036, 5.911) (41.7994, 5.9946) knots 0 0 0 1 1 1
  spline S43 degree 2 poles (41.7994, 5.9946) (41.6044, 6.0781) (41.3816, 6.0781) knots 0 0 0 1 1 1
  spline S44 degree 2 poles (41.3816, 6.0781) (41.1495, 6.0781) (40.9452, 5.9946) knots 0 0 0 1 1 1
  spline S45 degree 2 poles (40.9452, 5.9946) (40.7503, 5.911) (40.6017, 5.7625) knots 0 0 0 1 1 1
  spline S46 degree 2 poles (40.6017, 5.7625) (40.4625, 5.6139) (40.3789, 5.419) knots 0 0 0 1 1 1
  spline S47 degree 2 poles (40.3789, 5.419) (40.2954, 5.2333) (40.2954, 5.0105) knots 0 0 0 1 1 1
  line L7 (42.4121, 7.3779) -> (44.1017, 7.3779)
  line L8 (44.1017, 7.3779) -> (44.1017, 2.6153)
  line L9 (44.1017, 2.6153) -> (42.4121, 2.6153)
  line L10 (42.4121, 2.6153) -> (42.4121, 3.1444)
  spline S48 degree 2 poles (42.4121, 3.1444) (41.8736, 2.4667) (40.9545, 2.4667) knots 0 0 0 1 1 1
  spline S49 degree 2 poles (40.9545, 2.4667) (40.4346, 2.4667) (39.9983, 2.6524) knots 0 0 0 1 1 1
  spline S50 degree 2 poles (39.9983, 2.6524) (39.562, 2.8474) (39.237, 3.1909) knots 0 0 0 1 1 1
  spline S51 degree 2 poles (39.237, 3.1909) (38.9121, 3.5344) (38.7264, 3.9985) knots 0 0 0 1 1 1
  spline S52 degree 2 poles (38.7264, 3.9985) (38.55, 4.4627) (38.55, 5.0105) knots 0 0 0 1 1 1
  spline S53 degree 2 poles (38.55, 5.0105) (38.55, 5.5211) (38.7264, 5.976) knots 0 0 0 1 1 1
  spline S54 degree 2 poles (38.7264, 5.976) (38.9028, 6.4402) (39.2185, 6.7837) knots 0 0 0 1 1 1
  spline S55 degree 2 poles (39.2185, 6.7837) (39.5341, 7.1272) (39.9704, 7.3222) knots 0 0 0 1 1 1
  spline S56 degree 2 poles (39.9704, 7.3222) (40.4068, 7.5264) (40.936, 7.5264) knots 0 0 0 1 1 1
  spline S57 degree 2 poles (40.936, 7.5264) (41.8272, 7.5264) (42.4121, 6.9044) knots 0 0 0 1 1 1
  line L11 (42.4121, 6.9044) -> (42.4121, 7.3779)
  line L12 (46.924, 10.3208) -> (46.924, 2.6153)
  line L13 (46.924, 2.6153) -> (45.2436, 2.6153)
  line L14 (45.2436, 2.6153) -> (45.2436, 10.3208)
  line L15 (45.2436, 10.3208) -> (46.924, 10.3208)
  spline S58 degree 2 poles (69.3688, 7.4102) (68.7375, 8.1808) (67.8091, 8.1808) knots 0 0 0 1 1 1
  spline S59 degree 2 poles (67.8091, 8.1808) (67.4007, 8.1808) (67.0479, 8.0322) knots 0 0 0 1 1 1
  spline S60 degree 2 poles (67.0479, 8.0322) (66.7044, 7.8837) (66.4537, 7.6237) knots 0 0 0 1 1 1
  spline S61 degree 2 poles (66.4537, 7.6237) (66.203, 7.3731) (66.0545, 7.0203) knots 0 0 0 1 1 1
  spline S62 degree 2 poles (66.0545, 7.0203) (65.9152, 6.6675) (65.9152, 6.259) knots 0 0 0 1 1 1
  spline S63 degree 2 poles (65.9152, 6.259) (65.9152, 5.8412) (66.0545, 5.4885) knots 0 0 0 1 1 1
  spline S64 degree 2 poles (66.0545, 5.4885) (66.203, 5.1357) (66.4537, 4.8757) knots 0 0 0 1 1 1
  spline S65 degree 2 poles (66.4537, 4.8757) (66.7137, 4.6158) (67.0572, 4.4672) knots 0 0 0 1 1 1
  spline S66 degree 2 poles (67.0572, 4.4672) (67.4007, 4.3187) (67.7999, 4.3187) knots 0 0 0 1 1 1
  spline S67 degree 2 poles (67.7999, 4.3187) (68.6725, 4.3187) (69.3688, 5.0614) knots 0 0 0 1 1 1
  line L16 (69.3688, 5.0614) -> (69.3688, 2.9076)
  line L17 (69.3688, 2.9076) -> (69.1831, 2.8426)
  spline S68 degree 2 poles (69.1831, 2.8426) (68.7654, 2.694) (68.4033, 2.629) knots 0 0 0 1 1 1
  spline S69 degree 2 poles (68.4033, 2.629) (68.0412, 2.5548) (67.6885, 2.5548) knots 0 0 0 1 1 1
  spline S70 degree 2 poles (67.6885, 2.5548) (66.9643, 2.5548) (66.2959, 2.824) knots 0 0 0 1 1 1
  spline S71 degree 2 poles (66.2959, 2.824) (65.6367, 3.1025) (65.1261, 3.5946) knots 0 0 0 1 1 1
  spline S72 degree 2 poles (65.1261, 3.5946) (64.6248, 4.0959) (64.3184, 4.7736) knots 0 0 0 1 1 1
  spline S73 degree 2 poles (64.3184, 4.7736) (64.0121, 5.4606) (64.0121, 6.2683) knots 0 0 0 1 1 1
  spline S74 degree 2 poles (64.0121, 6.2683) (64.0121, 7.076) (64.3091, 7.7444) knots 0 0 0 1 1 1
  spline S75 degree 2 poles (64.3091, 7.7444) (64.6155, 8.4221) (65.1168, 8.9049) knots 0 0 0 1 1 1
  spline S76 degree 2 poles (65.1168, 8.9049) (65.6274, 9.397) (66.2959, 9.6662) knots 0 0 0 1 1 1
  spline S77 degree 2 poles (66.2959, 9.6662) (66.9643, 9.9447) (67.6977, 9.9447) knots 0 0 0 1 1 1
  spline S78 degree 2 poles (67.6977, 9.9447) (68.1155, 9.9447) (68.5147, 9.8519) knots 0 0 0 1 1 1
  spline S79 degree 2 poles (68.5147, 9.8519) (68.9232, 9.7683) (69.3688, 9.5826) knots 0 0 0 1 1 1
  line L18 (69.3688, 9.5826) -> (69.3688, 7.4102)
  line L19 (72.0426, 7.5123) -> (72.0426, 2.7497)
  line L20 (72.0426, 2.7497) -> (70.3622, 2.7497)
  line L21 (70.3622, 2.7497) -> (70.3622, 7.5123)
  line L22 (70.3622, 7.5123) -> (72.0426, 7.5123)
  spline S80 degree 2 poles (70.2508, 9.3412) (70.2508, 9.5362) (70.3251, 9.7033) knots 0 0 0 1 1 1
  spline S81 degree 2 poles (70.3251, 9.7033) (70.3993, 9.8797) (70.5293, 10.0097) knots 0 0 0 1 1 1
  spline S82 degree 2 poles (70.5293, 10.0097) (70.6593, 10.1397) (70.8264, 10.2139) knots 0 0 0 1 1 1
  spline S83 degree 2 poles (70.8264, 10.2139) (71.0028, 10.2882) (71.1977, 10.2882) knots 0 0 0 1 1 1
  spline S84 degree 2 poles (71.1977, 10.2882) (71.3927, 10.2882) (71.5598, 10.2139) knots 0 0 0 1 1 1
  spline S85 degree 2 poles (71.5598, 10.2139) (71.7362, 10.1397) (71.8662, 10.0097) knots 0 0 0 1 1 1
  spline S86 degree 2 poles (71.8662, 10.0097) (71.9961, 9.8797) (72.0704, 9.7033) knots 0 0 0 1 1 1
  spline S87 degree 2 poles (72.0704, 9.7033) (72.1447, 9.5362) (72.1447, 9.3412) knots 0 0 0 1 1 1
  spline S88 degree 2 poles (72.1447, 9.3412) (72.1447, 9.1463) (72.0704, 8.9699) knots 0 0 0 1 1 1
  spline S89 degree 2 poles (72.0704, 8.9699) (71.9961, 8.8028) (71.8662, 8.6728) knots 0 0 0 1 1 1
  spline S90 degree 2 poles (71.8662, 8.6728) (71.7362, 8.5428) (71.5598, 8.4686) knots 0 0 0 1 1 1
  spline S91 degree 2 poles (71.5598, 8.4686) (71.3927, 8.3943) (71.1977, 8.3943) knots 0 0 0 1 1 1
  spline S92 degree 2 poles (71.1977, 8.3943) (71.0028, 8.3943) (70.8264, 8.4686) knots 0 0 0 1 1 1
  spline S93 degree 2 poles (70.8264, 8.4686) (70.6593, 8.5428) (70.5293, 8.6728) knots 0 0 0 1 1 1
  spline S94 degree 2 poles (70.5293, 8.6728) (70.3993, 8.8028) (70.3251, 8.9699) knots 0 0 0 1 1 1
  spline S95 degree 2 poles (70.3251, 8.9699) (70.2508, 9.1463) (70.2508, 9.3412) knots 0 0 0 1 1 1
  line L23 (73.1938, 7.5123) -> (74.8741, 7.5123)
  line L24 (74.8741, 7.5123) -> (74.8741, 6.7325)
  spline S96 degree 2 poles (74.8741, 6.7325) (75.1434, 7.1596) (75.5333, 7.3824) knots 0 0 0 1 1 1
  spline S97 degree 2 poles (75.5333, 7.3824) (75.9232, 7.6145) (76.4431, 7.6145) knots 0 0 0 1 1 1
  spline S98 degree 2 poles (76.4431, 7.6145) (76.5081, 7.6145) (76.5824, 7.6145) knots 0 0 0 1 1 1
  spline S99 degree 2 poles (76.5824, 7.6145) (76.6659, 7.6145) (76.768, 7.5959) knots 0 0 0 1 1 1
  line L25 (76.768, 7.5959) -> (76.768, 5.9898)
  spline S100 degree 2 poles (76.768, 5.9898) (76.4338, 6.1569) (76.0439, 6.1569) knots 0 0 0 1 1 1
  spline S101 degree 2 poles (76.0439, 6.1569) (75.459, 6.1569) (75.1619, 5.8041) knots 0 0 0 1 1 1
  spline S102 degree 2 poles (75.1619, 5.8041) (74.8741, 5.4606) (74.8741, 4.7922) knots 0 0 0 1 1 1
  line L26 (74.8741, 4.7922) -> (74.8741, 2.7497)
  line L27 (74.8741, 2.7497) -> (73.1938, 2.7497)
  line L28 (73.1938, 2.7497) -> (73.1938, 7.5123)
  spline S103 degree 2 poles (81.1036, 5.9712) (80.6672, 6.2683) (80.2216, 6.2683) knots 0 0 0 1 1 1
  spline S104 degree 2 poles (80.2216, 6.2683) (79.9802, 6.2683) (79.7667, 6.1847) knots 0 0 0 1 1 1
  spline S105 degree 2 poles (79.7667, 6.1847) (79.5625, 6.1012) (79.4046, 5.9434) knots 0 0 0 1 1 1
  spline S106 degree 2 poles (79.4046, 5.9434) (79.2468, 5.7948) (79.154, 5.5813) knots 0 0 0 1 1 1
  spline S107 degree 2 poles (79.154, 5.5813) (79.0704, 5.3771) (79.0704, 5.1171) knots 0 0 0 1 1 1
  spline S108 degree 2 poles (79.0704, 5.1171) (79.0704, 4.8664) (79.154, 4.6529) knots 0 0 0 1 1 1
  spline S109 degree 2 poles (79.154, 4.6529) (79.2468, 4.4487) (79.3953, 4.2908) knots 0 0 0 1 1 1
  spline S110 degree 2 poles (79.3953, 4.2908) (79.5532, 4.1423) (79.7667, 4.0588) knots 0 0 0 1 1 1
  spline S111 degree 2 poles (79.7667, 4.0588) (79.9802, 3.9752) (80.2216, 3.9752) knots 0 0 0 1 1 1
  spline S112 degree 2 poles (80.2216, 3.9752) (80.6951, 3.9752) (81.1036, 4.3001) knots 0 0 0 1 1 1
  line L29 (81.1036, 4.3001) -> (81.1036, 2.8704)
  spline S113 degree 2 poles (81.1036, 2.8704) (80.4816, 2.6012) (79.9245, 2.6012) knots 0 0 0 1 1 1
  spline S114 degree 2 poles (79.9245, 2.6012) (79.4046, 2.6012) (78.9312, 2.7776) knots 0 0 0 1 1 1
  spline S115 degree 2 poles (78.9312, 2.7776) (78.467, 2.954) (78.1049, 3.2789) knots 0 0 0 1 1 1
  spline S116 degree 2 poles (78.1049, 3.2789) (77.7521, 3.6131) (77.5386, 4.068) knots 0 0 0 1 1 1
  spline S117 degree 2 poles (77.5386, 4.068) (77.3251, 4.5322) (77.3251, 5.0985) knots 0 0 0 1 1 1
  spline S118 degree 2 poles (77.3251, 5.0985) (77.3251, 5.6649) (77.5293, 6.129) knots 0 0 0 1 1 1
  spline S119 degree 2 poles (77.5293, 6.129) (77.7335, 6.6025) (78.0863, 6.9367) knots 0 0 0 1 1 1
  spline S120 degree 2 poles (78.0863, 6.9367) (78.4391, 7.2802) (78.9219, 7.4659) knots 0 0 0 1 1 1
  spline S121 degree 2 poles (78.9219, 7.4659) (79.4139, 7.6609) (79.9709, 7.6609) knots 0 0 0 1 1 1
  spline S122 degree 2 poles (79.9709, 7.6609) (80.5837, 7.6609) (81.1036, 7.4009) knots 0 0 0 1 1 1
  line L30 (81.1036, 7.4009) -> (81.1036, 5.9712)
  line L31 (83.7402, 10.4553) -> (83.7402, 2.7497)
  line L32 (83.7402, 2.7497) -> (82.0598, 2.7497)
  line L33 (82.0598, 2.7497) -> (82.0598, 10.4553)
  line L34 (82.0598, 10.4553) -> (83.7402, 10.4553)
  spline S123 degree 2 poles (88.3728, 5.8227) (88.2892, 6.1755) (88.0293, 6.389) knots 0 0 0 1 1 1
  spline S124 degree 2 poles (88.0293, 6.389) (87.7694, 6.6025) (87.398, 6.6025) knots 0 0 0 1 1 1
  spline S125 degree 2 poles (87.398, 6.6025) (87.0081, 6.6025) (86.7574, 6.3983) knots 0 0 0 1 1 1
  spline S126 degree 2 poles (86.7574, 6.3983) (86.516, 6.194) (86.451, 5.8227) knots 0 0 0 1 1 1
  line L35 (86.451, 5.8227) -> (88.3728, 5.8227)
  spline S127 degree 2 poles (86.4046, 4.8479) (86.4046, 3.7617) (87.4259, 3.7617) knots 0 0 0 1 1 1
  spline S128 degree 2 poles (87.4259, 3.7617) (87.9736, 3.7617) (88.2521, 4.2073) knots 0 0 0 1 1 1
  line L36 (88.2521, 4.2073) -> (89.8768, 4.2073)
  spline S129 degree 2 poles (89.8768, 4.2073) (89.3847, 2.5733) (87.4166, 2.5733) knots 0 0 0 1 1 1
  spline S130 degree 2 poles (87.4166, 2.5733) (86.8131, 2.5733) (86.3118, 2.7497) knots 0 0 0 1 1 1
  spline S131 degree 2 poles (86.3118, 2.7497) (85.8105, 2.9354) (85.4484, 3.2696) knots 0 0 0 1 1 1
  spline S132 degree 2 poles (85.4484, 3.2696) (85.0956, 3.6038) (84.9007, 4.068) knots 0 0 0 1 1 1
  spline S133 degree 2 poles (84.9007, 4.068) (84.7057, 4.5322) (84.7057, 5.1078) knots 0 0 0 1 1 1
  spline S134 degree 2 poles (84.7057, 5.1078) (84.7057, 5.702) (84.8914, 6.1755) knots 0 0 0 1 1 1
  spline S135 degree 2 poles (84.8914, 6.1755) (85.077, 6.6582) (85.4205, 6.9924) knots 0 0 0 1 1 1
  spline S136 degree 2 poles (85.4205, 6.9924) (85.764, 7.3267) (86.2468, 7.5031) knots 0 0 0 1 1 1
  spline S137 degree 2 poles (86.2468, 7.5031) (86.7388, 7.6887) (87.3516, 7.6887) knots 0 0 0 1 1 1
  spline S138 degree 2 poles (87.3516, 7.6887) (87.955, 7.6887) (88.4378, 7.5031) knots 0 0 0 1 1 1
  spline S139 degree 2 poles (88.4378, 7.5031) (88.9205, 7.3267) (89.2548, 6.9832) knots 0 0 0 1 1 1
  spline S140 degree 2 poles (89.2548, 6.9832) (89.589, 6.6397) (89.7654, 6.1383) knots 0 0 0 1 1 1
  spline S141 degree 2 poles (89.7654, 6.1383) (89.9418, 5.6463) (89.9418, 5.0243) knots 0 0 0 1 1 1
  line L37 (89.9418, 5.0243) -> (89.9418, 4.8479)
  line L38 (89.9418, 4.8479) -> (86.4046, 4.8479)
hidden bodies 1 5
named bodies: "OLED_acrylic", "keyplate", "backplate", "OLED_circle_window", "OLED_oval_window"
